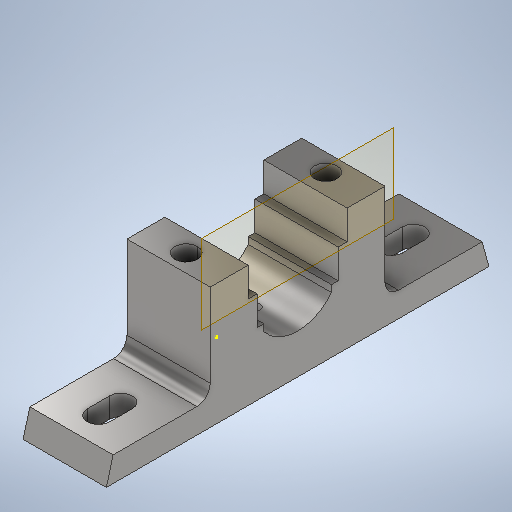
# Autodesk Inventor part: base
Saved by Autodesk Inventor 2025.2 (Build 292293000, 293)
## iProperties
Created: 2025-04-15
Part Number: base
Material: Iron, Malleable
Document SubType Name: Modeling
Designer: bless
Density: 7.15 g/cm^3
Appearance: Semi-Polished
Author: bless
Autodesk Inventor part; units mm, degrees
ref_plane "YZ Plane" through (0, 0, 0) normal (1, 0, 0) x (0, 1, 0)
ref_plane "XZ Plane" through (0, 0, 0) normal (0, 1, 0) x (-1, 0, 0)
ref_plane "XY Plane" through (0, 0, 0) normal (0, 0, 1) x (1, 0, 0)
ref_plane "Work Plane1" through (21.3568, 20.7673, 2.7504) normal (1, 0, 0) x (0, 1, 0)
sketch "Sketch1" plane through (21.3568, 20.7673, 2.7504) normal (1, 0, 0) x (0, 1, 0)
  point P0 (-20.7673, -2.7504)
sketch "Sketch2" plane through (21.3568, 20.7673, 2.7504) normal (1, 0, 0) x (0, 1, 0)
  line L0 (0, 0) -> (0, -16.8188) projected
  line L1 (0, -16.8188) -> (-13, -16.8188) projected
  line L2 (-13, -16.8188) -> (-13, -20.7888) projected
  arc A0 (-13, -56.8488) -> (-13, -20.7888) centre (-19.0031, -38.8188) ccw projected
  line L3 (-13, -56.8488) -> (-13, -60.8188) projected
  line L4 (-13, -60.8188) -> (0, -60.8188) projected
  line L5 (0, -60.8188) -> (0, -77.6375) projected
  line L6 (0, -77.6375) -> (10, -77.6375) projected
  line L7 (10, -63.4021) -> (10, -77.6375) projected
  arc A1 (10, -63.4021) -> (10, -14.2354) centre (-19.0031, -38.8188) ccw projected
  line L8 (10, 0) -> (10, -14.2354) projected
  line L9 (0, 0) -> (10, 0) projected
  line L10 (0, -16.8188) -> (-13, -16.8188)
  line L11 (-13, -20.7888) -> (-13, -16.8188)
  line L12 (-13, -16.8188) -> (0, -16.8188)
  line L13 (0, 0) -> (-37, 0)
  line L14 (-43, 6) -> (-43, 43.1812)
  line L15 (-43, 43.1812) -> (-54, 46.1812)
  line L16 (-13, -56.8488) -> (-13, -60.8188)
  line L17 (0, -60.8188) -> (0, -77.6375)
  line L18 (-13, -56.8488) -> (-13, -60.8188)
  line L19 (-13, -60.8188) -> (0, -60.8188)
  line L20 (0, -60.8188) -> (0, -77.6375)
  line L21 (0, -77.6375) -> (-37, -77.6375)
  line L22 (-43, -83.6375) -> (-43, -120.8188)
  line L23 (-43, -120.8188) -> (-54, -123.8188)
  line L24 (-54, 46.1812) -> (-54, -123.8188)
  arc A2 (-43, 6) -> (-37, 0) centre (-37, 6) ccw
  arc A3 (-37, -77.6375) -> (-43, -83.6375) centre (-37, -83.6375) ccw
  line L25 (-13, -20.7888) -> (-26, -20.7888)
  line L26 (-26, -20.7888) -> (-26, -23.7888)
  line L27 (-26, -23.7888) -> (-29, -23.7888)
  line L28 (-13, -56.8488) -> (-26, -56.8488)
  line L29 (-26, -56.8488) -> (-26, -53.8488)
  line L30 (-26, -53.8488) -> (-29, -53.8488)
  arc A4 (-29, -23.7888) -> (-29, -53.8488) centre (-17.3768, -38.8188) ccw
  point P0 (-20.7673, -2.7504)
  point P1 (0, -38.8188)
  point P2 (-54, -38.8188)
  point P3 (0, -8.4094)
  dimension "d0" = 170
  dimension "d1" = 43
  dimension "d2" = 43
  dimension "d5" = 11
  dimension "d6" = 6
  dimension "d7" = 6
  dimension "d8" = 3
  dimension "d9" = 3
  dimension "d11" = 13
  dimension "d12" = 3
  dimension "d13" = 3
  dimension "d14" = 13
  dimension "d15" = 3
  dimension "d16" = 3
  dimension "d17" = 19
  constraints: 42 end point, 8 collinear, 7 point on circle, 4 horizontal, 4 perpendicular, 4 tangent, 3 centre point, 3 vertical, 2 midpoint, 1 horizontal alignment
  measures "d0" distance of L15.end L23.end
  measures "d1" distance between parallel lines of L22 L5
  measures "d2" distance from line of L14 point (0, -8.409)
  measures "d5" distance between parallel lines of L24 L14
  measures "d6" radius of A2
  measures "d7" radius of A3
  measures "d8" vertical distance of L14.end L15.end
  measures "d9" vertical distance of L23.end L22.end
  measures "d11" distance of L2.end L25.end
  measures "d12" distance of L25.end L26.end
  measures "d13" distance of L26.end L27.end
  measures "d14" distance of L3.start L28.end
  measures "d15" distance of L28.end L29.end
  measures "d16" distance of L29.end L30.end
  measures "d17" radius of A4
extrude "Extrusion1" add sketch "Sketch2" against normal blind 37 contours L0 L1 L2 L25 L26 L27 A4 L30 L29 L28 L3 L4 L5 L21 A3 L22 L23 L24 L15 L14 A2 L13
sketch "Sketch3" plane through (21.3568, -33.2327, -121.0684) normal (0, -1, 0) x (1, 0, 0)
  line L0 (0, 170) -> (-37, 170) projected
  line L1 (-37, 0) -> (-37, 170) projected
  line L2 (0, 0) -> (-37, 0) projected
  line L3 (-7.5, 160) -> (-29.5, 160)
  line L4 (-29.5, 160) -> (-29.5, 89)
  line L5 (-29.5, 89) -> (-7.5, 89)
  line L6 (-7.5, 89) -> (-7.5, 160)
  line L7 (-7.5, 160) -> (-29.5, 89) construction
  line L8 (-29.5, 160) -> (-7.5, 89) construction
  line L9 (-7.5, 81) -> (-29.5, 81)
  line L10 (-29.5, 81) -> (-29.5, 10)
  line L11 (-29.5, 10) -> (-7.5, 10)
  line L12 (-7.5, 10) -> (-7.5, 81)
  line L13 (-7.5, 81) -> (-29.5, 10) construction
  line L14 (-29.5, 81) -> (-7.5, 10) construction
  point P0 (-21.3568, 121.0684)
  point P1 (-18.5, 124.5)
  point P2 (-18.5, 45.5)
  dimension "d20" = 22
  dimension "d21" = 71
  dimension "d22" = 22
  dimension "d23" = 71
  dimension "d24" = 10
  dimension "d25" = 10
  dimension "d26" = 7.5
  dimension "d27" = 7.5
  constraints: 24 end point, 4 midpoint, 4 parallel, 2 horizontal, 2 perpendicular
  measures "d20" distance of L5.end L4.end
  measures "d21" distance of L4.end L3.end
  measures "d22" distance of L11.end L10.end
  measures "d23" distance of L10.end L9.end
  measures "d24" distance between parallel lines of L3 L0
  measures "d25" distance between parallel lines of L11 L2
  measures "d26" distance between parallel lines of L1 L4
  measures "d27" distance between parallel lines of L1 L10
extrude "Extrusion2" cut sketch "Sketch3" against normal blind 2
sketch "Sketch4" plane through (21.3568, -31.2327, -121.0684) normal (0, -1, 0) x (1, 0, 0)
  line L0 (-7.5, 160) -> (-7.5, 89) projected
  circle A0 centre (-18.5, 116) radius 5
  line L1 (-8.5, 126) -> (-28.5, 126)
  line L2 (-28.5, 126) -> (-28.5, 106)
  line L3 (-28.5, 106) -> (-8.5, 106)
  line L4 (-8.5, 106) -> (-8.5, 126)
  line L5 (-8.5, 126) -> (-28.5, 106) construction
  line L6 (-28.5, 126) -> (-8.5, 106) construction
  arc A1 (-13.5, 155) -> (-23.5, 155) centre (-18.5, 155) ccw
  line L7 (-29.5, 160) -> (-7.5, 160) projected
  arc A2 (-23.5, 145) -> (-13.5, 145) centre (-18.5, 145) ccw
  line L8 (-13.5, 155) -> (-13.5, 145)
  line L9 (-23.5, 145) -> (-23.5, 155)
  line L10 (-29.5, 10) -> (-29.5, 81) projected
  line L11 (-7.5, 10) -> (-29.5, 10) projected
  line L12 (-7.5, 81) -> (-7.5, 10) projected
  line L13 (-29.5, 81) -> (-7.5, 81) projected
  circle A3 centre (-18.4961, 116) radius 5 projected
  circle A4 centre (-18.4961, 54) radius 5 projected
  circle A5 centre (-18.4961, 54) radius 5
  line L14 (-8.4961, 64) -> (-28.4961, 64)
  line L15 (-28.4961, 64) -> (-28.4961, 44)
  line L16 (-28.4961, 44) -> (-8.4961, 44)
  line L17 (-8.4961, 44) -> (-8.4961, 64)
  line L18 (-8.4961, 64) -> (-28.4961, 44) construction
  line L19 (-28.4961, 64) -> (-8.4961, 44) construction
  arc A6 (-23.5, 15) -> (-13.5, 15) centre (-18.5, 15) ccw
  line L20 (-7.5, 10) -> (-29.5, 10) projected
  arc A7 (-13.5, 25) -> (-23.5, 25) centre (-18.5, 25) ccw
  line L21 (-13.5, 15) -> (-13.5, 25)
  line L22 (-23.5, 15) -> (-23.5, 25)
  point P0 (-21.3568, 121.0684)
  point P1 (-16.4961, 85)
  point P2 (-18.498, 121)
  point P3 (-18.498, 111)
  dimension "d30" = 10
  dimension "d31" = 20
  dimension "d33" = 5
  dimension "d34" = 5
  dimension "d35" = 0
  dimension "d36" = 20
  dimension "d37" = 1
  dimension "d38" = 6
  dimension "d39" = 20
  dimension "d40" = 20
  dimension "d41" = 5
  dimension "d42" = 5
  dimension "d43" = 6
  constraints: 32 end point, 10 tangent, 8 point on circle, 6 centre point, 6 parallel, 4 midpoint, 2 horizontal, 2 perpendicular, 1 coincident, 1 concentric, 1 other
  measures "d30" diameter of A0
  measures "d31" distance of L3.end L2.end
  measures "d33" radius of A1
  measures "d34" radius of A2
  measures "d35" vertical distance of A3.centre A0.centre
  measures "d36" distance of L1.end L2.end
  measures "d37" distance between parallel lines of L0 L4
  measures "d38" distance between parallel lines of L0 L8
  measures "d39" distance of L16.end L15.end
  measures "d40" distance of L15.end L14.end
  measures "d41" radius of A6
  measures "d42" radius of A7
  measures "d43" distance between parallel lines of L21 L12
extrude "Extrusion3" cut sketch "Sketch4" against normal through all contours A0 A3 | A0 A3 | A3 A0 | L8 A2 L9 A1 | A6 L22 A7 L21 | A4
sketch "Sketch5" plane through (21.3568, -31.2327, -121.0684) normal (0, -1, 0) x (1, 0, 0)
  arc A0 (-18.498, 121) -> (-18.498, 111) centre (-18.4961, 116) ccw projected
  arc A1 (-18.498, 111) -> (-18.498, 121) centre (-18.5, 116) ccw projected
  line L0 (-8.5, 126) -> (-28.5, 126)
  line L1 (-28.5, 126) -> (-28.5, 106)
  line L2 (-28.5, 106) -> (-8.5, 106)
  line L3 (-8.5, 106) -> (-8.5, 126)
  line L4 (-8.5, 126) -> (-28.5, 106) construction
  line L5 (-28.5, 126) -> (-8.5, 106) construction
  line L6 (-8.4961, 64) -> (-28.4961, 64)
  line L7 (-28.4961, 64) -> (-28.4961, 44)
  line L8 (-28.4961, 44) -> (-8.4961, 44)
  line L9 (-8.4961, 44) -> (-8.4961, 64)
  circle A2 centre (-18.4961, 54) radius 5 projected
  line L10 (-8.4961, 64) -> (-28.4961, 44) construction
  line L11 (-28.4961, 64) -> (-8.4961, 44) construction
  point P0 (-21.3568, 121.0684)
  dimension "d46" = 20
  dimension "d47" = 20
  dimension "d48" = 20
  dimension "d49" = 20
  constraints: 24 end point, 4 midpoint, 4 parallel, 2 horizontal, 2 perpendicular
  measures "d46" distance of L2.end L1.end
  measures "d47" distance of L1.end L0.end
  measures "d48" distance of L8.end L7.end
  measures "d49" distance of L7.end L6.end
extrude "Extrusion4" cut sketch "Sketch5" against normal blind 4
sketch "Sketch6" plane through (21.3568, -33.2327, -121.0684) normal (0, -1, 0) x (1, 0, 0)
  spline S0 degree 3 poles (-18.4961, 87) (-18.7472, 87) (-19.0151, 86.9498) (-19.5079, 86.7457) (-19.7327, 86.5918) (-20.0878, 86.2367) (-20.2417, 86.0118) (-20.4459, 85.5191) (-20.4961, 85.2512) (-20.4961, 84.7488) (-20.4459, 84.4809) (-20.2417, 83.9882) (-20.0878, 83.7633) (-19.7327, 83.4082) (-19.5079, 83.2543) (-19.0151, 83.0502) (-18.7472, 83) (-18.2449, 83) (-17.977, 83.0502) (-17.4843, 83.2543) (-17.2594, 83.4082) (-16.9043, 83.7633) (-16.7504, 83.9882) (-16.5463, 84.4809) (-16.4961, 84.7488) (-16.4961, 85.2512) (-16.5463, 85.5191) (-16.7504, 86.0118) (-16.9043, 86.2367) (-17.2594, 86.5918) (-17.4843, 86.7457) (-17.977, 86.9498) (-18.2449, 87) (-18.4961, 87) knots 0 0 0 0 0.075352 0.075352 0.150705 0.150705 0.226057 0.226057 0.301409 0.301409 0.376761 0.376761 0.452114 0.452114 0.527466 0.527466 0.602818 0.602818 0.67817 0.67817 0.753523 0.753523 0.828875 0.828875 0.904227 0.904227 0.979579 0.979579 1.054932 1.054932 1.130284 1.130284 1.205636 1.205636 1.205636 1.205636 projected
  point P0 (-21.3568, 121.0684)
  point P1 (-18.4961, 87)
extrude "Extrusion5" cut sketch "Sketch6" against normal up to surface round surface about axis through (21.3568, 3.3905, -36.0684) along (-1, 0, 0) radius 19 far side no
sketch "Sketch7" plane through (21.3568, -33.2327, -121.0684) normal (0, -1, 0) x (1, 0, 0)
  spline S0 degree 3 poles (-18.4961, 87) (-18.7472, 87) (-19.0151, 86.9498) (-19.5079, 86.7457) (-19.7327, 86.5918) (-20.0878, 86.2367) (-20.2417, 86.0118) (-20.4459, 85.5191) (-20.4961, 85.2512) (-20.4961, 84.7488) (-20.4459, 84.4809) (-20.2417, 83.9882) (-20.0878, 83.7633) (-19.7327, 83.4082) (-19.5079, 83.2543) (-19.0151, 83.0502) (-18.7472, 83) (-18.2449, 83) (-17.977, 83.0502) (-17.4843, 83.2543) (-17.2594, 83.4082) (-16.9043, 83.7633) (-16.7504, 83.9882) (-16.5463, 84.4809) (-16.4961, 84.7488) (-16.4961, 85.2512) (-16.5463, 85.5191) (-16.7504, 86.0118) (-16.9043, 86.2367) (-17.2594, 86.5918) (-17.4843, 86.7457) (-17.977, 86.9498) (-18.2449, 87) (-18.4961, 87) knots 0 0 0 0 0.0625 0.0625 0.125 0.125 0.1875 0.1875 0.25 0.25 0.3125 0.3125 0.375 0.375 0.4375 0.4375 0.5 0.5 0.5625 0.5625 0.625 0.625 0.6875 0.6875 0.75 0.75 0.8125 0.8125 0.875 0.875 0.9375 0.9375 1 1 1 1 projected
  point P0 (-21.3568, 121.0684)
  constraints: 1 other
extrude "Extrusion6" add sketch "Sketch7" against normal blind 11.623
body "Solid1"
